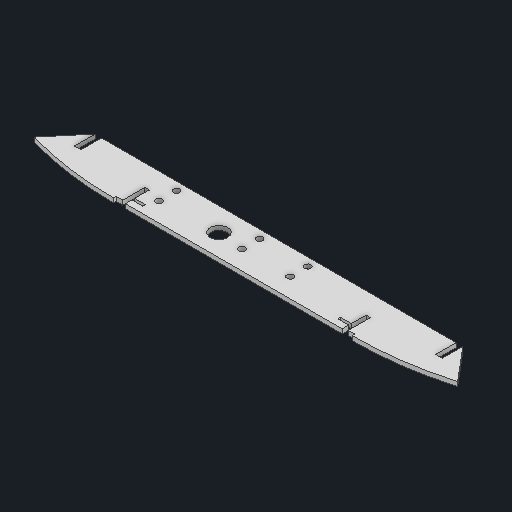
# Autodesk Inventor part: transom
Saved by Autodesk Inventor 2023 (Build 270158030, 158C)
## iProperties
Created: 2022-03-21
Part Number: transom
Material: Generic
Document SubType Name: Modeling
Designer: kardo
Density: 1 g/cm^3
Appearance: Default
Author: kardo
Autodesk Inventor part; units mm, degrees
ref_plane "YZ Plane" through (0, 0, 0) normal (1, 0, 0) x (0, 1, 0)
ref_plane "XZ Plane" through (0, 0, 0) normal (0, 1, 0) x (-1, 0, 0)
ref_plane "XY Plane" through (0, 0, 0) normal (0, 0, 1) x (1, 0, 0)
derived "parameters_frame.ipt"
derived "stencil_frame.ipt"
sketch "sk_joint_locations" plane through (81.12, 0, 0) normal (1, 0, 0) x (0, 1, 0)
  line L0 (0, 0) -> (122.4, 8.559) construction
  line L1 (36.465, 28.832) -> (112.2, 28.832) construction
  arc A0 (36.465, 28.832) -> (11.22, 28.376) centre (36.465, -670.197) ccw construction
  line L2 (-241.5001, 19.2432) -> (11.22, 28.376) construction
  line L3 (-345, 16.32) -> (-262.2001, 18.586) construction
  arc A1 (-262.2001, 18.586) -> (-241.5001, 19.2432) centre (-326.8578, 2381.2399) ccw construction
  line L4 (-95.1358, 3119.4657) -> (254.2444, -1876.9042) construction
  line L5 (-230.0001, 3089.1136) -> (-230.0001, -1866.0023) construction
  line L6 (-114.9999, 3089.1136) -> (-114.9999, -1866.0023) construction
  line L7 (-345, 3089.1136) -> (-345, -1866.0023) construction
  line L8 (0, 3089.1136) -> (0, -1866.0023) construction
  line L9 (516.4305, 45.5774) -> (-594.5903, 6.7797) construction
  line L10 (-657.7604, -27.3784) -> (621.8174, 62.0984) construction
  line L11 (193.4506, 30.2962) -> (193.1714, 38.2913) construction
  line L12 (201.1621, 36.7028) -> (201.7215, 28.7028) construction
  line L13 (0, 14.96) -> (121.9304, 15.2746) construction
  line L14 (-230.0001, 45.8702) -> (-230.0001, 19.6588) construction
  line L15 (-345, 37.4554) -> (-345, 16.32) construction
  line L16 (-114.9999, 51.0173) -> (-114.9999, 23.8147) construction
  line L17 (0, 52.89) -> (0, 27.9705) construction
  line L18 (119.462, 50.575) -> (119.9556, 43.5149) construction
  line L19 (120.4493, 36.4549) -> (119.9556, 43.5149) construction
  line L20 (120.4493, 36.4549) -> (120.943, 29.3948) construction
  line L21 (120.943, 29.3948) -> (121.4367, 22.3347) construction
  line L22 (121.4367, 22.3347) -> (121.9304, 15.2746) construction
  line L23 (0, 14.96) -> (0, 0) construction
  spline S0 degree 4 poles (-345, 37.4554) (-258.8682, 45.1562) (-172.5926, 49.7838) (-86.3161, 52.89) (0, 52.89) knots 0 0 0 0 0 1 1 1 1 1
  spline S1 degree 3 poles (0, 52.89) (92.8353, 52.89) (195.0311, 49.5089) (255, 36.448) knots 0 0 0 0 1 1 1 1
  spline S2 degree 2 poles (122.4, 8.559) (190.3044, 13.3074) (255, 36.448) knots 0 0 0 1 1 1
  line L24 (112.2, 37.536) -> (112.2, 28.832) construction
  line L25 (112.2, 35.548) -> (112.2, 30.82) construction
  point P0 (-95.1358, 3119.4657)
  point P1 (254.2444, -1876.9042)
  point P2 (193.311, 34.2938)
  point P3 (201.4418, 32.7028)
  point P4 (134.9575, 11.3411)
  point P5 (-345, 26.8877)
  point P6 (-230.0001, 32.7645)
  point P7 (-114.9999, 37.416)
  point P8 (0, 40.4303)
  point P9 (112.2, 33.184)
sketch "sk_rudder_mount" plane through (0, -345, 0) normal (0, 1, 0) x (-1, 0, 0)
  line L0 (54.6, -1866.0023) -> (54.6, 3089.1136) construction
  line L1 (0, 16.32) -> (54.6, 16.32) construction
  line L2 (43, 29.32) -> (43, 21.32) construction
  point P0 (0, 0)
  point P1 (0, 39.712)
sketch3d "sk_servo_rod"
sketch "sk_cowl_joint_locations" plane through (54.6, 0, 0) normal (1, 0, 0) x (0, 1, 0)
  line L0 (-345, 16.32) -> (-262.2001, 18.586) construction
  arc A0 (-262.2001, 18.586) -> (-241.5001, 19.2432) centre (-326.8578, 2381.2399) ccw construction
  line L1 (-241.5001, 19.2432) -> (11.22, 28.376) construction
  arc A1 (36.465, 28.832) -> (11.22, 28.376) centre (36.465, -670.197) ccw construction
  line L2 (36.465, 28.832) -> (112.2, 28.832) construction
  line L3 (94.8, 30.032) -> (36.465, 30.032) construction
  arc A2 (36.465, 30.032) -> (11.1767, 29.5752) centre (36.465, -670.197) ccw construction
  line L4 (11.1767, 29.5752) -> (-241.5434, 20.4424) construction
  arc A3 (-262.2329, 19.7855) -> (-241.5434, 20.4424) centre (-326.8578, 2381.2399) ccw construction
  line L5 (-262.2329, 19.7855) -> (-345, 17.5204) construction
  line L6 (-230.0001, 3089.1136) -> (-230.0001, -1866.0023) construction
  line L7 (-114.9999, 3089.1136) -> (-114.9999, -1866.0023) construction
  line L8 (-345, 3089.1136) -> (-345, -1866.0023) construction
  line L9 (0, 3089.1136) -> (0, -1866.0023) construction
  line L10 (-230.0001, 45.0685) -> (-230.0001, 20.8596) construction
  line L11 (-114.9999, 49.9659) -> (-114.9999, 25.0155) construction
  line L12 (-345, 17.5204) -> (-345, 17.5204)
  line L13 (-345, 17.5204) -> (-345, 36.9221) construction
  line L14 (-869.78, 3004.1953) -> (348.339, -1881.413) construction
  line L15 (-344.7623, 36.9221) -> (-345, 39.712) construction
  line L16 (0, 51.6) -> (0, 29.1713) construction
  spline S0 degree 2 poles (-345, 39.712) (-172.656, 54.3934) (0, 54.4) knots 0 0 0 1 1 1
  spline S1 degree 3 poles (0, 54.4) (37.026, 54.4) (80.784, 47.9917) (112.2, 37.536) knots 1 1 1 1 2 2 2 2
  spline S2 degree 3 poles (111.3158, 34.8793) (106.1488, 36.5989) (96.4909, 39.4217) (84.5445, 42.2265) (75.2974, 44.1359) (69.0059, 45.3094) (61.0256, 46.6466) (54.5653, 47.6105) (46.4371, 48.6777) (39.9092, 49.4192) (31.7597, 50.2005) (25.2653, 50.7072) (17.2211, 51.1873) (9.2717, 51.5118) (3.0586, 51.6) (0, 51.6) knots 1 1 1 1 1.166667 1.291667 1.333333 1.416667 1.458333 1.541667 1.583333 1.666667 1.708333 1.791667 1.833333 1.916667 2 2 2 2
  spline S3 degree 3 poles (0, 51.6) (-19.1708, 51.5993) (-52.7146, 51.3604) (-91.0402, 50.6121) (-119.7801, 49.8472) (-138.9379, 49.2354) (-162.8824, 48.3434) (-182.0358, 47.528) (-205.975, 46.3814) (-225.1241, 45.3623) (-249.0578, 43.9611) (-268.2026, 42.7383) (-292.131, 41.0825) (-316.0566, 39.2994) (-335.1942, 37.7372) (-344.7623, 36.9221) knots 0 0 0 0 0.166667 0.291667 0.333333 0.416667 0.458333 0.541666 0.583333 0.666666 0.708333 0.791666 0.833333 0.916666 1 1 1 1
  line L17 (-136.2088, 45.4676) -> (-130.9657, 24.4385) construction
  line L18 (-128.3953, 30.6635) -> (-132.2764, 29.6958) construction
  line L19 (-131.0168, 41.178) -> (-134.898, 40.2103) construction
  line L20 (-136.2088, 45.4676) -> (-132.3276, 46.4353) construction
  line L21 (-130.9657, 24.4385) -> (-127.0845, 25.4062) construction
  line L22 (-132.3276, 46.4353) -> (-132.5171, 52.2322) construction
  point P0 (0, 0)
  point P1 (-345, 27.2213)
  point P2 (-230.0001, 32.964)
  point P3 (-114.9999, 37.4907)
  point P4 (0, 40.3857)
  point P5 (-869.78, 3004.1953)
  point P6 (348.339, -1881.413)
  point P7 (-85.2629, 50.788)
  point P8 (0, 40.3857)
sketch "sk_strut_mount" plane through (0, -345, 0) normal (0, 1, 0) x (-1, 0, 0)
  line L0 (-6, -1866.0023) -> (-6, 3089.1136) construction
  line L1 (5, 21.32) -> (-17, 21.32) construction
  line L2 (5, 29.32) -> (-17, 29.32) construction
  line L3 (5, 21.32) -> (5, 29.32) construction
  line L4 (-17, 29.32) -> (-17, 21.32) construction
  point P0 (0, 0)
  point P1 (0, 39.712)
  point P2 (0, 16.32)
  point P3 (-6, 29.32)
  point P4 (-6, 21.32)
sketch "sk_transom_base" plane through (0, -345, 0) normal (0, 1, 0) x (-1, 0, 0)
  line L0 (-54.6, 39.712) -> (0, 39.712) construction
  spline S0 degree 2 poles (-54.6, 39.712) (-110.5674, 39.712) (-156, 1.324) knots 0 0 0 1 1 1 construction
  line L1 (0, -1280.4843) -> (0, 2991.5273) construction
  line L2 (-54.6, -1280.4843) -> (-54.6, 2991.5273) construction
  line L3 (-81.12, -1280.4843) -> (-81.12, 2991.5273) construction
  line L4 (-1606.1721, 1829.4544) -> (672.974, -886.7262) construction
  line L5 (-96.8398, 32.569) -> (-84.12, 17.4101)
  line L6 (-84.12, 17.4101) -> (-84.12, 26.8877)
  line L7 (-84.12, 26.8877) -> (-81.12, 26.8877)
  line L8 (-81.12, 26.8877) -> (-81.12, 17.52)
  line L9 (-81.12, 17.52) -> (0, 17.52)
  line L10 (0, 38.112) -> (0, 17.52)
  line L11 (-54.6, 38.512) -> (-54.6, 38.112)
  line L12 (-54.6, 38.112) -> (0, 38.112)
  spline S1 degree 5 poles (-54.6, 38.512) (-65.4115, 38.5116) (-76.222, 37.6116) (-86.9353, 35.72) (-108.2158, 29.8227) (-128.0428, 20.0839) (-137.6309, 14.2233) (-146.6864, 7.6225) (-155.2255, 0.4074) knots 0 0 0 0 0 0 0.491644 0.491644 0.491644 1 1 1 1 1 1
  point P0 (0, 0)
  point P1 (-34.32, 16.32)
  dimension "d3" = 1.2
  dimension "d2" = 1.2
  dimension "d4" = 3
  dimension "d5" = 1.2
  dimension "d36" = 1.6
  constraints: 16 end point, 3 perpendicular, 2 collinear, 2 parallel, 2 point on line, 4 other
  measures "d2" distance between parallel lines of L4 L5
  measures "d4" distance of L6.end L7.end
  measures "d5" distance from line of L9 point (-34.32, 16.32)
  measures "d36" distance between parallel lines of L0 L12
extrude "thicken" add sketch "sk_transom_base" along normal blind 2
sketch "sk_cut_joint" plane through (0, -345, 0) normal (0, 1, 0) x (-1, 0, 0)
  line L0 (-54.6, 39.712) -> (0, 39.712) projected
  line L1 (-54.6, -1280.4843) -> (-54.6, 2991.5273) construction
  line L2 (-49.6, 39.712) -> (-49.6, 27.2213)
  line L3 (-49.6, 27.2213) -> (-51.6, 27.2213)
  line L4 (-51.6, 27.2213) -> (-51.6, 39.712)
  point P0 (0, 0)
  point P1 (-54.6, 27.2213)
  dimension "d25" = 2
  dimension "d26" = 5
  constraints: 6 end point, 3 parallel, 3 point on line
  measures "d25" distance between parallel lines of L2 L4
  measures "d26" distance between parallel lines of L2 L1
extrude "cut_joint" cut sketch "sk_cut_joint" along normal through all both and the other way through all
sketch "sk_cut_liner" plane through (0, -345, 0) normal (0, 1, 0) x (-1, 0, 0)
  line L0 (-54.6, 39.712) -> (0, 39.712) construction
  line L1 (-54.6, -1280.4843) -> (-54.6, 2991.5273) projected
  line L2 (-44.6, 39.712) -> (-44.6, 33.912)
  line L3 (-44.6, 33.912) -> (-49.6, 33.912)
  line L4 (-49.6, 33.912) -> (-49.6, 37.312)
  line L5 (-49.6, 37.312) -> (-54.6, 37.312)
  line L6 (-44.6, 35.112) -> (-49.6, 35.112)
  line L7 (-49.6, 39.712) -> (-49.6, 37.312)
  line L8 (-49.6, 39.712) -> (-54.6, 39.712)
  point P0 (0, 0)
  dimension "d29" = 5
  dimension "d30" = 5
  dimension "d32" = 2.4
  dimension "d33" = 1.2
  dimension "d37" = 5.8
  constraints: 14 end point, 6 parallel, 5 point on line
  measures "d29" distance between parallel lines of L1 L4
  measures "d30" distance between parallel lines of L4 L2
  measures "d32" distance between parallel lines of L0 L5
  measures "d33" distance between parallel lines of L3 L6
  measures "d37" distance between parallel lines of L0 L3
extrude "cut_liner" cut sketch "sk_cut_liner" along normal through all both and the other way through all
mirror "mirror" about plane through (0, 0, 0) normal (1, 0, 0)
hole "drill_rudder" at (-43, -345, 29.32) at (-43, -345, 21.32) direction (0, 1, 0) diameter 3 end through all
sketch "sk_servo_rod_drill" plane through (0, -345, 0) normal (0, 1, 0) x (-1, 0, 0)
  line L0 (15.288, 28.1324) -> (16.768, 28.1324) construction
  line L1 (0, -1280.4843) -> (0, 2991.5273) construction
  point P0 (0, 0)
  dimension "d38" = 1.48
  constraints: 2 end point, 1 coincident, 1 perpendicular
  measures "d38" distance of L0.start L0.end
hole "drill_servo_rod" at (-16.768, -345, 28.1324) direction (0, 1, 0) diameter 8 end through all
hole "Hole4" at (-5, -345, 29.32) at (17, -345, 29.32) at (17, -345, 21.32) at (-5, -345, 21.32) direction (0, 1, 0) diameter 3 end through all
equation "\"d3\" = shell_thickness"
equation "\"d2\" = shell_thickness"
equation "\"d4\" = stringer_thickness"
equation "\"d5\" = shell_thickness"
equation "\"d36\" = cowl_shell_thickness"
equation "\"d7\" = bulkhead_thickness"
equation "\"d25\" = bulkhead_thickness"
equation "\"d26\" = cowl_liner_width"
equation "\"d29\" = cowl_liner_width"
equation "\"d30\" = cowl_sealing_width"
equation "\"d32\" = shell_thickness + cowl_liner_thickness"
equation "\"d33\" = cowl_liner_thickness"
equation "\"d37\" = cowl_sealing_thickness + cowl_shell_thickness + cowl_liner_thickness"
equation "\"d9\" = drill_rudder_mount_diam"
equation "\"d38\" = 0.185 * drill_servo_rod_diam"
equation "\"d39\" = drill_servo_rod_diam"
equation "\"d46\" = drill_struct_mount_diam"
equation "\"shell_thickness\" = 1.2"
equation "\"stringer_thickness\" = 3"
equation "\"cowl_shell_thickness\" = 1.6"
equation "\"bulkhead_thickness\" = 2"
equation "\"cowl_liner_width\" = 5"
equation "\"cowl_sealing_width\" = 5"
equation "\"cowl_liner_thickness\" = 1.2"
equation "\"cowl_sealing_thickness\" = 3"
equation "\"drill_rudder_mount_diam\" = 3"
equation "\"drill_servo_rod_diam\" = 8"
equation "\"drill_struct_mount_diam\" = 3"
body "Solid1"
